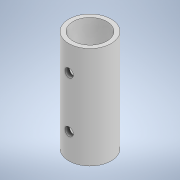
# Autodesk Inventor part: airfoil
Saved by Autodesk Inventor 2022 (Build 260153000, 153)
## iProperties
Created: 2021-03-06
Part Number: airfoil
Material: Generic
Document SubType Name: Modeling
Designer: Ferdinand Hubbard
Density: 1 g/cm^3
Appearance: Default
Author: Ferdinand Hubbard
Autodesk Inventor part; units mm, degrees
ref_plane "YZ Plane" through (0, 0, 0) normal (1, 0, 0) x (0, 1, 0)
ref_plane "XZ Plane" through (0, 0, 0) normal (0, 1, 0) x (-1, 0, 0)
ref_plane "XY Plane" through (0, 0, 0) normal (0, 0, 1) x (1, 0, 0)
sketch "Sketch9" plane through (0, 0, 0) normal (0, 1, 0) x (-1, 0, 0)
  circle A0 centre (0, 0) radius 4
  circle A1 centre (0, 0) radius 5
  dimension "d140" = 8
  dimension "d149" = 10
  constraints: 2 centre point, 2 coincident
  measures "d140" diameter of A0
  measures "d149" diameter of A1
extrude "Extrusion10" add sketch "Sketch9" along normal blind 24
sketch "Sketch10" plane through (0, 0, 0) normal (0, 0, 1) x (1, 0, 0)
  line L0 (0, 0) -> (0, 6)
  circle A0 centre (0, 6) radius 1
  line L1 (-4, 24) -> (4, 24) projected
  line L2 (0, 24) -> (0, 18)
  circle A1 centre (0, 18) radius 1
  dimension "d143" = 6
  dimension "d144" = 2
  dimension "d145" = 6
  dimension "d146" = 2
  constraints: 4 end point, 2 centre point, 2 coincident, 2 vertical, 1 midpoint
  measures "d143" distance of L0.start L0.end
  measures "d144" diameter of A0
  measures "d145" distance of L2.start L2.end
  measures "d146" diameter of A1
extrude "Extrusion11" cut sketch "Sketch10" along normal mid plane 24
body "Solid8"
